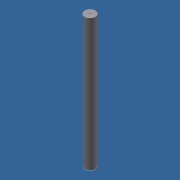
# Autodesk Inventor part: P1704_005_guideRessort
Saved by Autodesk Inventor 2019 (Build 230136000, 136)
## iProperties
Created: 2019-04-30
Part Number: P1704_005_guideRessort
Project: Nom Projet
Material: .
Description: Nom pièce
Document SubType Name: Modeling
Designer: Joan.MAILLARD
Authority: brut Ø
Density: 0.001 g/cm^3
Appearance: Par défaut
Author: Joan.MAILLARD
Material number: ---
Autodesk Inventor part; units mm, degrees
ref_plane "Plan YZ" through (0, 0, 0) normal (1, 0, 0) x (0, 1, 0)
ref_plane "Plan XZ" through (0, 0, 0) normal (0, 1, 0) x (-1, 0, 0)
ref_plane "Plan XY" through (0, 0, 0) normal (0, 0, 1) x (1, 0, 0)
sketch "Esquisse1" plane through (0, 0, 0) normal (0, 0, 1) x (1, 0, 0)
  point P0 (0, 0)
sketch "Esquisse6" plane through (0, 0, 0) normal (0, 1, 0) x (-1, 0, 0)
  line L0 (0.0412, -0.002) -> (1.5412, -0.002)
  line L1 (1.5412, -0.002) -> (1.5412, -38.002)
  line L2 (1.5412, -38.002) -> (0.0412, -38.002)
  line L3 (0.0412, -38.002) -> (0.0412, -0.002)
  dimension "d0" = 1.5
  dimension "d1" = 38
  constraints: 8 end point, 2 parallel, 1 horizontal, 1 perpendicular
  measures "d0" distance of L1.end L2.end
  measures "d1" distance of L0.end L1.end
revolve "Révolution1" add sketch "Esquisse6" angle 360 about axis through (-0.0412, 0, -38.002) along (0, 0, 1)
